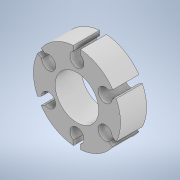
# Autodesk Inventor part: Beschleuniger_Hub
Saved by Autodesk Inventor 2021 (Build 250183000, 183)
## iProperties
Created: 2024-01-21
Part Number: Beschleuniger_Hub
Material: Generic
Document SubType Name: Modeling
Designer: Lukas
Density: 1 g/cm^3
Appearance: Default
Author: Lukas
Autodesk Inventor part; units mm, degrees
ref_plane "YZ Plane" through (0, 0, 0) normal (1, 0, 0) x (0, 1, 0)
ref_plane "XZ Plane" through (0, 0, 0) normal (0, 1, 0) x (-1, 0, 0)
ref_plane "XY Plane" through (0, 0, 0) normal (0, 0, 1) x (1, 0, 0)
sketch "Sketch1" plane through (0, 0, 0) normal (0, 0, 1) x (1, 0, 0)
  circle A0 centre (0, 0) radius 5
  circle A1 centre (0, 0) radius 10
  arc A2 (-0.8, 8.8856) -> (0.8, 8.8856) centre (0, 7.5) ccw
  line L0 (-0.8, 8.8856) -> (-0.8, 10)
  line L1 (-0.8, 10) -> (0.8, 10)
  line L2 (0.8, 10) -> (0.8, 8.8856)
  arc A3 (-8.0952, 3.75) -> (-7.2952, 5.1356) centre (-6.4952, 3.75) ccw
  line L3 (-8.0952, 3.75) -> (-9.0603, 4.3072)
  line L4 (-9.0603, 4.3072) -> (-8.2603, 5.6928)
  line L5 (-8.2603, 5.6928) -> (-7.2952, 5.1356)
  arc A4 (-7.2952, -5.1356) -> (-8.0952, -3.75) centre (-6.4952, -3.75) ccw
  line L6 (-7.2952, -5.1356) -> (-8.2603, -5.6928)
  line L7 (-8.2603, -5.6928) -> (-9.0603, -4.3072)
  line L8 (-9.0603, -4.3072) -> (-8.0952, -3.75)
  arc A5 (0.8, -8.8856) -> (-0.8, -8.8856) centre (0, -7.5) ccw
  line L9 (0.8, -8.8856) -> (0.8, -10)
  line L10 (0.8, -10) -> (-0.8, -10)
  line L11 (-0.8, -10) -> (-0.8, -8.8856)
  arc A6 (8.0952, -3.75) -> (7.2952, -5.1356) centre (6.4952, -3.75) ccw
  line L12 (8.0952, -3.75) -> (9.0603, -4.3072)
  line L13 (9.0603, -4.3072) -> (8.2603, -5.6928)
  line L14 (8.2603, -5.6928) -> (7.2952, -5.1356)
  arc A7 (7.2952, 5.1356) -> (8.0952, 3.75) centre (6.4952, 3.75) ccw
  line L15 (7.2952, 5.1356) -> (8.2603, 5.6928)
  line L16 (8.2603, 5.6928) -> (9.0603, 4.3072)
  line L17 (9.0603, 4.3072) -> (8.0952, 3.75)
  point P0 (-0.8, 9.9679)
  point P1 (-8.2325, 5.6768)
  point P2 (-9.0325, 4.2912)
  point P3 (-9.0325, -4.2912)
  point P4 (-8.2325, -5.6768)
  point P5 (-0.8, -9.9679)
  point P6 (0.8, -9.9679)
  point P7 (8.2325, -5.6768)
  point P8 (9.0325, -4.2912)
  point P9 (9.0325, 4.2912)
  point P10 (8.2325, 5.6768)
  point P11 (0.8, 9.9679)
  dimension "d0" = 10
  dimension "d4" = 20
  dimension "d6" = 7.5
  dimension "d7" = 1.6
  dimension "d8" = 1.6
  dimension "d11" = 360
  constraints: 36 end point, 12 point on circle, 8 centre point, 4 coincident, 2 vertical, 1 horizontal alignment, 1 perpendicular, 1 tangent, 1 vertical alignment, 55 other
  measures "d0" diameter of A0
  measures "d4" diameter of A1
  measures "d6" distance of point (0, 0) A2.centre
  measures "d7" distance between parallel lines of L2 L0
  measures "d8" radius of A2
extrude "Extrusion1" add sketch "Sketch1" along normal blind 6 contours A1 L12 A6 L14 L9 A5 L11 L6 A4 L8 L3 A3 L5 L0 A2 L2 L15 A7 L17
equation "\"d6\" = 0.25 * d4 + 0.25 * d0"
body "Solid1"
